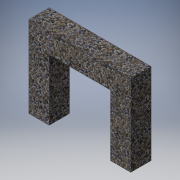
# Autodesk Inventor part: RailsMini2
Saved by Autodesk Inventor 2016 (Build 200138000, 138)
## iProperties
Created: 2015-08-17
Part Number: RailsMini2
Material: Concrete
Document SubType Name: Modeling
Designer: myhome
Mass: 26480.4 g
Surface Area: 4600 cm^2
Volume: 11000 cm^3
Density: 2.40731 g/cm^3
Appearance: Exposed Aggregate - Coarse
Author: myhome
Autodesk Inventor part; units mm, degrees
ref_plane "YZ Plane" through (0, 0, 0) normal (1, 0, 0) x (0, 1, 0)
ref_plane "XZ Plane" through (0, 0, 0) normal (0, 1, 0) x (-1, 0, 0)
ref_plane "XY Plane" through (0, 0, 0) normal (0, 0, 1) x (1, 0, 0)
sketch "Sketch1" plane through (0, 0, 0) normal (0, 0, 1) x (1, 0, 0)
  line L0 (0, 0) -> (100, 0)
  line L1 (0, 0) -> (0, 400)
  line L2 (0, 400) -> (500, 400)
  line L3 (500, 400) -> (500, 0)
  line L4 (500, 0) -> (400, 0)
  line L5 (400, 0) -> (400, 300)
  line L6 (400, 300) -> (100, 300)
  line L7 (100, 300) -> (100, 0)
  dimension "d0" = 100
  dimension "d1" = 400
  dimension "d2" = 500
  dimension "d3" = 400
  dimension "d4" = 100
  dimension "d5" = 300
  dimension "d6" = 300
  dimension "d7" = 300
  constraints: 16 end point, 5 perpendicular, 1 horizontal, 1 vertical
  measures "d0" distance of L0.start L0.end
  measures "d1" distance of L0.start L1.end
  measures "d2" distance of L1.end L2.end
  measures "d3" distance of L2.end L3.end
  measures "d4" distance of L3.end L4.end
  measures "d5" distance of L4.end L5.end
  measures "d6" distance of L5.end L6.end
  measures "d7" distance of L6.end L0.end
extrude "Extrusion1" add sketch "Sketch1" against normal blind 100
body "Solid1"
